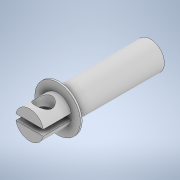
# Autodesk Inventor part: pole
Saved by Autodesk Inventor 2021 (Build 250183000, 183)
## iProperties
Created: 2020-06-26
Part Number: pole
Material: Generic
Document SubType Name: Modeling
Designer: Yatekii
Density: 1 g/cm^3
Appearance: Default
Author: Yatekii
Autodesk Inventor part; units mm, degrees
ref_plane "YZ Plane" through (0, 0, 0) normal (1, 0, 0) x (0, 1, 0)
ref_plane "XZ Plane" through (0, 0, 0) normal (0, 1, 0) x (-1, 0, 0)
ref_plane "XY Plane" through (0, 0, 0) normal (0, 0, 1) x (1, 0, 0)
sketch "Sketch2" plane through (0, 0, 0) normal (1, 0, 0) x (0, 1, 0)
  line L0 (0, 21.8412) -> (4, 21.8412)
  line L1 (4, 21.8412) -> (4, 13.8412)
  line L2 (4, 13.8412) -> (6.5, 13.8412)
  line L3 (6.5, 13.8412) -> (6.5, 13.3412)
  line L4 (6.5, 13.3412) -> (4, 13.3412)
  line L5 (4, 13.3412) -> (4, -12.6588)
  line L6 (4, -12.6588) -> (0, -12.6588)
  line L7 (0, -12.6588) -> (0, 21.8412)
  point P0 (0, 0)
  dimension "d0" = 4
  dimension "d1" = 8
  dimension "d2" = 2.5
  dimension "d3" = 0.5
  dimension "d4" = 26
  constraints: 16 end point, 5 perpendicular, 1 horizontal, 1 parallel, 1 vertical
  measures "d0" distance of L0.start L0.end
  measures "d1" distance of L0.end L1.end
  measures "d2" distance of L1.end L2.end
  measures "d3" distance of L2.end L3.end
  measures "d4" distance of L4.end L5.end
revolve "Revolution1" add sketch "Sketch2" angle 360 about axis through (0, 0, -12.6588) along (0, 0, 1)
sketch "Sketch3" plane through (0, 0, 21.8412) normal (0, 0, 1) x (1, 0, 0)
  line L0 (5.071, -0.8298) -> (-5.071, -0.8298)
  line L1 (-5.071, -0.8298) -> (-5.071, 0.8298)
  line L2 (-5.071, 0.8298) -> (5.071, 0.8298)
  line L3 (5.071, 0.8298) -> (5.071, -0.8298)
  circle A0 centre (0, 0) radius 4 projected
  line L4 (5.071, -0.8298) -> (-5.071, 0.8298) construction
  line L5 (-5.071, -0.8298) -> (5.071, 0.8298) construction
  point P0 (3.913, 0.8298)
  point P1 (-3.913, 0.8298)
  point P2 (-3.913, -0.8298)
  point P3 (3.913, -0.8298)
  constraints: 12 end point, 2 midpoint, 2 parallel, 1 horizontal, 1 perpendicular
extrude "Extrusion1" cut sketch "Sketch3" against normal blind 8 contours L0 A0 L2
sketch "Sketch5" plane through (-3.913, -0.8298, 21.8412) normal (0, 1, 0) x (1, 0, 0)
  circle A0 centre (3.913, 4) radius 2.3908
  line L0 (7.826, 0) -> (0, 0) projected
  line L1 (7.826, 0) -> (0, 0) projected
  line L2 (7.826, 0) -> (0, 0) projected
  line L3 (7.826, 8) -> (7.826, 0) projected
  line L4 (7.826, 0) -> (0, 0) projected
  line L5 (0, 0) -> (0, 8) projected
  line L6 (7.826, 8) -> (0, 8) projected
  point P0 (3.913, 21.8412)
  dimension "d8" = 4
  dimension "d9" = 3.913
  dimension "d10" = 3.913
  constraints: 1 centre point
  measures "d8" distance from line of L0 A0.centre
  measures "d9" distance from line of L3 A0.centre
  measures "d10" distance from line of L5 A0.centre
extrude "Extrusion2" cut sketch "Sketch5" along normal through all both and the other way through all contours A0
equation "\"d9\" = d10"
body "Solid1"
